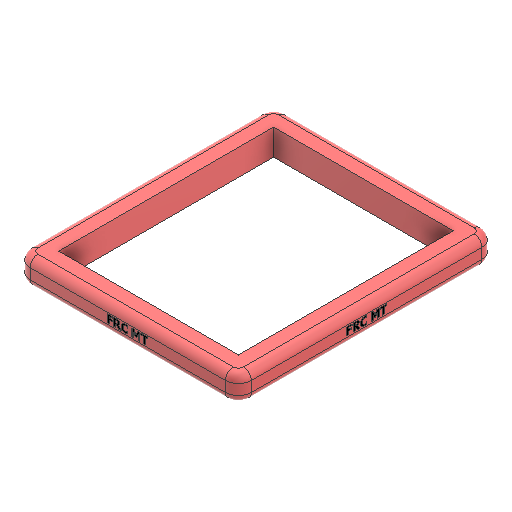
# Autodesk Inventor part: Bumper
Saved by Autodesk Inventor 2027.1 (Build 311270010, 270A)
## iProperties
Created: 2026-08-13
Part Number: Bumper
Material: Genérico
Document SubType Name: Modeling
Designer: djair.oliveira
Density: 1 g/cm^3
Appearance: Padrão
Author: djair.oliveira
Autodesk Inventor part; units mm, degrees
ref_plane "YZ Plane" through (0, 0, 0) normal (1, 0, 0) x (0, 1, 0)
ref_plane "XZ Plane" through (0, 0, 0) normal (0, 1, 0) x (-1, 0, 0)
ref_plane "XY Plane" through (0, 0, 0) normal (0, 0, 1) x (1, 0, 0)
sketch "Esboço1" plane through (0, 0, 0) normal (0, 1, 0) x (-1, 0, 0)
  line L0 (-346.4954, -410.2857) -> (343.3046, -410.2857)
  line L1 (343.3046, -410.2857) -> (343.3046, 414.3883)
  line L2 (343.3046, 414.3883) -> (-346.4954, 414.3883)
  line L3 (-346.4954, 414.3883) -> (-346.4954, -410.2857)
  line L4 (373.3046, -490.2857) -> (-376.4954, -490.2857)
  line L5 (-426.4954, -440.2857) -> (-426.4954, 444.3883)
  line L6 (-376.4954, 494.3883) -> (373.3046, 494.3883)
  line L7 (423.3046, 444.3883) -> (423.3046, -440.2857)
  arc A0 (373.3046, -490.2857) -> (423.3046, -440.2857) centre (373.3046, -440.2857) ccw
  arc A1 (423.3046, 444.3883) -> (373.3046, 494.3883) centre (373.3046, 444.3883) ccw
  arc A2 (-376.4954, 494.3883) -> (-426.4954, 444.3883) centre (-376.4954, 444.3883) ccw
  arc A3 (-426.4954, -440.2857) -> (-376.4954, -490.2857) centre (-376.4954, -440.2857) ccw
  point P0 (0, 0)
  dimension "d4" = 80
  dimension "d5" = 50
  constraints: 16 end point, 8 point on circle, 8 tangent, 4 centre point, 4 parallel, 3 equal radius, 2 perpendicular, 1 horizontal, 3 other
  measures "d4" distance between parallel lines of L0 L4
  measures "d5" radius of A0
extrude "Extrusão1" add sketch "Esboço1" along normal blind 100
fillet "Arredondamento1" radius 30 16 edges at (-408.6599, 100, 479.7436) (1.5954, 100, 494.3883) (411.8508, 100, 479.7436) (426.4954, 100, 2.0513) (411.8508, 100, -475.6411) (1.5954, 100, -490.2857) (-408.6599, 100, -475.6411) (-423.3046, 100, 2.0513) (411.8508, 0, -475.6411) (1.5954, 0, -490.2857) (-408.6599, 0, -475.6411) (-423.3046, 0, 2.0513) (-408.6599, 0, 479.7436) (1.5954, 0, 494.3883) (411.8508, 0, 479.7436) (426.4954, 0, 2.0513)
sketch "Esboço2" plane through (426.4954, 30, -440.2857) normal (1, 0, 0) x (0, 0, -1)
  line L0 (-521.7524, 35.8457) -> (-358.819, 35.8457) construction
  line L1 (-358.819, 35.8457) -> (-358.819, 4.1543) construction
  line L2 (-358.819, 4.1543) -> (-521.7524, 4.1543) construction
  line L3 (-521.7524, 4.1543) -> (-521.7524, 35.8457) construction
  line L4 (-498.5595, 29.5491) -> (-511.1527, 29.5491)
  line L5 (-511.1527, 29.5491) -> (-511.1527, 23.8846)
  line L6 (-511.1527, 23.8846) -> (-499.5563, 23.8846)
  line L7 (-499.5563, 23.8846) -> (-499.5563, 18.1715)
  line L8 (-499.5563, 18.1715) -> (-511.1527, 18.1715)
  line L9 (-511.1527, 18.1715) -> (-511.1527, 5.2623)
  line L10 (-511.1527, 5.2623) -> (-518.6406, 5.2623)
  line L11 (-518.6406, 5.2623) -> (-518.6406, 35.2623)
  line L12 (-518.6406, 35.2623) -> (-498.5595, 35.2623)
  line L13 (-498.5595, 35.2623) -> (-498.5595, 29.5491)
  line L14 (-466.955, 5.2623) -> (-476.1203, 5.2623)
  line L15 (-476.1203, 5.2623) -> (-484.459, 16.2752)
  line L16 (-484.459, 16.2752) -> (-487.1819, 16.2752)
  line L17 (-487.1819, 16.2752) -> (-487.1819, 5.2623)
  line L18 (-487.1819, 5.2623) -> (-494.6697, 5.2623)
  line L19 (-494.6697, 5.2623) -> (-494.6697, 35.2623)
  line L20 (-494.6697, 35.2623) -> (-482.6114, 35.2623)
  spline S0 degree 2 poles (-482.6114, 35.2623) (-480.1073, 35.2623) (-476.412, 34.6302) (-474.8318, 33.6577) knots 0 0 0 1 2 2 2
  spline S1 degree 2 poles (-474.8318, 33.6577) (-473.2273, 32.6367) (-471.331, 29.4519) (-471.331, 27.0208) knots 0 0 0 1 2 2 2
  spline S2 degree 2 poles (-471.331, 27.0208) (-471.331, 23.5929) (-474.4428, 19.2898) (-477.0441, 18.0256) knots 0 0 0 1 2 2 2
  line L21 (-477.0441, 18.0256) -> (-466.955, 5.2623)
  spline S3 degree 2 poles (-479.062, 26.0726) (-479.062, 27.2153) (-479.9372, 28.8441) (-480.9339, 29.2817) knots 0 0 0 1 2 2 2
  spline S4 degree 2 poles (-480.9339, 29.2817) (-481.639, 29.5735) (-483.365, 29.7436) (-484.6535, 29.7436) knots 0 0 0 1 2 2 2
  line L22 (-484.6535, 29.7436) -> (-487.1819, 29.7436)
  line L23 (-487.1819, 29.7436) -> (-487.1819, 21.6723)
  line L24 (-487.1819, 21.6723) -> (-485.0182, 21.6723)
  spline S5 degree 2 poles (-485.0182, 21.6723) (-483.4623, 21.6723) (-481.25, 22.0613) (-480.4963, 22.6691) knots 0 0 0 1 2 2 2
  spline S6 degree 2 poles (-480.4963, 22.6691) (-479.767, 23.2525) (-479.062, 24.8085) (-479.062, 26.0726) knots 0 0 0 1 2 2 2
  spline S7 degree 2 poles (-451.7848, 4.6788) (-458.5433, 4.6788) (-466.4688, 12.8474) (-466.4688, 20.238) knots 0 0 0 1 2 2 2
  spline S8 degree 2 poles (-466.4688, 20.238) (-466.4688, 27.3611) (-458.519, 35.8457) (-451.7605, 35.8457) knots 0 0 0 1 2 2 2
  spline S9 degree 2 poles (-451.7605, 35.8457) (-449.9858, 35.8457) (-447.1171, 35.4324) (-445.8043, 35.0921) knots 0 0 0 1 2 2 2
  spline S10 degree 2 poles (-445.8043, 35.0921) (-444.7832, 34.776) (-442.3764, 33.7307) (-441.6227, 33.3417) knots 0 0 0 1 2 2 2
  line L25 (-441.6227, 33.3417) -> (-441.6227, 26.1942)
  line L26 (-441.6227, 26.1942) -> (-442.3764, 26.1942)
  spline S11 degree 2 poles (-442.3764, 26.1942) (-442.9355, 26.6804) (-444.5887, 28.0418) (-445.6341, 28.6739) knots 0 0 0 1 2 2 2
  spline S12 degree 2 poles (-445.6341, 28.6739) (-446.6795, 29.3303) (-449.1835, 30.2299) (-450.5693, 30.2299) knots 0 0 0 1 2 2 2
  spline S13 degree 2 poles (-450.5693, 30.2299) (-452.1981, 30.2299) (-454.8966, 29.2088) (-456.1365, 27.9203) knots 0 0 0 1 2 2 2
  spline S14 degree 2 poles (-456.1365, 27.9203) (-457.2548, 26.7777) (-458.6892, 22.8636) (-458.6892, 20.2136) knots 0 0 0 1 2 2 2
  spline S15 degree 2 poles (-458.6892, 20.2136) (-458.6892, 17.4179) (-457.2062, 13.601) (-455.9907, 12.4341) knots 0 0 0 1 2 2 2
  spline S16 degree 2 poles (-455.9907, 12.4341) (-454.8237, 11.2914) (-451.955, 10.2947) (-450.5206, 10.2947) knots 0 0 0 1 2 2 2
  spline S17 degree 2 poles (-450.5206, 10.2947) (-449.0377, 10.2947) (-446.3391, 11.2914) (-445.4153, 11.8992) knots 0 0 0 1 2 2 2
  spline S18 degree 2 poles (-445.4153, 11.8992) (-444.3942, 12.507) (-442.8626, 13.7955) (-442.3035, 14.306) knots 0 0 0 1 2 2 2
  line L27 (-442.3035, 14.306) -> (-441.6227, 14.306)
  line L28 (-441.6227, 14.306) -> (-441.6227, 7.2558)
  spline S19 degree 2 poles (-441.6227, 7.2558) (-442.4493, 6.8668) (-444.613, 5.8944) (-445.78, 5.554) knots 0 0 0 1 2 2 2
  spline S20 degree 2 poles (-445.78, 5.554) (-447.19, 5.1164) (-449.6454, 4.6788) (-451.7848, 4.6788) knots 0 0 0 1 2 2 2
  line L29 (-394.459, 5.2623) -> (-401.9469, 5.2623)
  line L30 (-401.9469, 5.2623) -> (-401.9469, 25.1488)
  line L31 (-401.9469, 25.1488) -> (-407.3926, 12.3125)
  line L32 (-407.3926, 12.3125) -> (-412.5466, 12.3125)
  line L33 (-412.5466, 12.3125) -> (-417.9923, 25.1488)
  line L34 (-417.9923, 25.1488) -> (-417.9923, 5.2623)
  line L35 (-417.9923, 5.2623) -> (-425.0911, 5.2623)
  line L36 (-425.0911, 5.2623) -> (-425.0911, 35.2623)
  line L37 (-425.0911, 35.2623) -> (-416.412, 35.2623)
  line L38 (-416.412, 35.2623) -> (-409.7508, 20.4568)
  line L39 (-409.7508, 20.4568) -> (-403.1381, 35.2623)
  line L40 (-403.1381, 35.2623) -> (-394.459, 35.2623)
  line L41 (-394.459, 35.2623) -> (-394.459, 5.2623)
  line L42 (-382.4736, 5.2623) -> (-382.4736, 29.5491)
  line L43 (-382.4736, 29.5491) -> (-391.3472, 29.5491)
  line L44 (-391.3472, 29.5491) -> (-391.3472, 35.2623)
  line L45 (-391.3472, 35.2623) -> (-366.0636, 35.2623)
  line L46 (-366.0636, 35.2623) -> (-366.0636, 29.5491)
  line L47 (-366.0636, 29.5491) -> (-374.9372, 29.5491)
  line L48 (-374.9372, 29.5491) -> (-374.9372, 5.2623)
  line L49 (-374.9372, 5.2623) -> (-382.4736, 5.2623)
  point P0 (-440.2857, -30)
  point P1 (-440.2857, 35.8457)
  point P2 (-358.819, 20)
  dimension "d9" = 0
  dimension "d10" = 50
  constraints: 2 midpoint, 2 other
  measures "d9" horizontal distance of point (-440.286, -30) point (-440.286, 35.846)
  measures "d10" vertical distance of point (-358.819, 20) point (-440.286, -30)
extrude "Extrusão2" cut sketch "Esboço2" against normal blind 0.1
sketch "Esboço3" plane through (376.4954, 30, -490.2857) normal (0, 0, -1) x (-1, 0, 0)
  line L0 (298.952, 35.0044) -> (454.0389, 35.0044) construction
  line L1 (454.0389, 35.0044) -> (454.0389, 4.9956) construction
  line L2 (454.0389, 4.9956) -> (298.952, 4.9956) construction
  line L3 (298.952, 4.9956) -> (298.952, 35.0044) construction
  line L4 (322.1449, 28.7078) -> (309.5517, 28.7078)
  line L5 (309.5517, 28.7078) -> (309.5517, 23.0433)
  line L6 (309.5517, 23.0433) -> (321.1481, 23.0433)
  line L7 (321.1481, 23.0433) -> (321.1481, 17.3301)
  line L8 (321.1481, 17.3301) -> (309.5517, 17.3301)
  line L9 (309.5517, 17.3301) -> (309.5517, 4.4209)
  line L10 (309.5517, 4.4209) -> (302.0638, 4.4209)
  line L11 (302.0638, 4.4209) -> (302.0638, 34.4209)
  line L12 (302.0638, 34.4209) -> (322.1449, 34.4209)
  line L13 (322.1449, 34.4209) -> (322.1449, 28.7078)
  line L14 (353.7494, 4.4209) -> (344.5841, 4.4209)
  line L15 (344.5841, 4.4209) -> (336.2454, 15.4339)
  line L16 (336.2454, 15.4339) -> (333.5225, 15.4339)
  line L17 (333.5225, 15.4339) -> (333.5225, 4.4209)
  line L18 (333.5225, 4.4209) -> (326.0347, 4.4209)
  line L19 (326.0347, 4.4209) -> (326.0347, 34.4209)
  line L20 (326.0347, 34.4209) -> (338.093, 34.4209)
  spline S0 degree 2 poles (338.093, 34.4209) (340.5971, 34.4209) (344.2924, 33.7888) (345.8726, 32.8164) knots 0 0 0 1 2 2 2
  spline S1 degree 2 poles (345.8726, 32.8164) (347.4771, 31.7953) (349.3734, 28.6105) (349.3734, 26.1794) knots 0 0 0 1 2 2 2
  spline S2 degree 2 poles (349.3734, 26.1794) (349.3734, 22.7515) (346.2616, 18.4485) (343.6603, 17.1843) knots 0 0 0 1 2 2 2
  line L21 (343.6603, 17.1843) -> (353.7494, 4.4209)
  spline S3 degree 2 poles (341.6425, 25.2313) (341.6425, 26.3739) (340.7673, 28.0028) (339.7705, 28.4404) knots 0 0 0 1 2 2 2
  spline S4 degree 2 poles (339.7705, 28.4404) (339.0655, 28.7321) (337.3394, 28.9023) (336.0509, 28.9023) knots 0 0 0 1 2 2 2
  line L22 (336.0509, 28.9023) -> (333.5225, 28.9023)
  line L23 (333.5225, 28.9023) -> (333.5225, 20.831)
  line L24 (333.5225, 20.831) -> (335.6862, 20.831)
  spline S5 degree 2 poles (335.6862, 20.831) (337.2421, 20.831) (339.4544, 21.2199) (340.2081, 21.8277) knots 0 0 0 1 2 2 2
  spline S6 degree 2 poles (340.2081, 21.8277) (340.9374, 22.4112) (341.6425, 23.9671) (341.6425, 25.2313) knots 0 0 0 1 2 2 2
  spline S7 degree 2 poles (368.9196, 3.8374) (362.1611, 3.8374) (354.2356, 12.006) (354.2356, 19.3966) knots 0 0 0 1 2 2 2
  spline S8 degree 2 poles (354.2356, 19.3966) (354.2356, 26.5198) (362.1854, 35.0044) (368.9439, 35.0044) knots 0 0 0 1 2 2 2
  spline S9 degree 2 poles (368.9439, 35.0044) (370.7186, 35.0044) (373.5873, 34.5911) (374.9002, 34.2507) knots 0 0 0 1 2 2 2
  spline S10 degree 2 poles (374.9002, 34.2507) (375.9212, 33.9347) (378.328, 32.8893) (379.0817, 32.5003) knots 0 0 0 1 2 2 2
  line L25 (379.0817, 32.5003) -> (379.0817, 25.3528)
  line L26 (379.0817, 25.3528) -> (378.328, 25.3528)
  spline S11 degree 2 poles (378.328, 25.3528) (377.7689, 25.8391) (376.1157, 27.2005) (375.0703, 27.8326) knots 0 0 0 1 2 2 2
  spline S12 degree 2 poles (375.0703, 27.8326) (374.0249, 28.489) (371.5209, 29.3885) (370.1352, 29.3885) knots 0 0 0 1 2 2 2
  spline S13 degree 2 poles (370.1352, 29.3885) (368.5063, 29.3885) (365.8078, 28.3674) (364.5679, 27.0789) knots 0 0 0 1 2 2 2
  spline S14 degree 2 poles (364.5679, 27.0789) (363.4496, 25.9363) (362.0152, 22.0222) (362.0152, 19.3723) knots 0 0 0 1 2 2 2
  spline S15 degree 2 poles (362.0152, 19.3723) (362.0152, 16.5765) (363.4982, 12.7596) (364.7138, 11.5927) knots 0 0 0 1 2 2 2
  spline S16 degree 2 poles (364.7138, 11.5927) (365.8807, 10.4501) (368.7494, 9.4533) (370.1838, 9.4533) knots 0 0 0 1 2 2 2
  spline S17 degree 2 poles (370.1838, 9.4533) (371.6668, 9.4533) (374.3653, 10.4501) (375.2891, 11.0579) knots 0 0 0 1 2 2 2
  spline S18 degree 2 poles (375.2891, 11.0579) (376.3102, 11.6656) (377.8418, 12.9541) (378.401, 13.4647) knots 0 0 0 1 2 2 2
  line L27 (378.401, 13.4647) -> (379.0817, 13.4647)
  line L28 (379.0817, 13.4647) -> (379.0817, 6.4144)
  spline S19 degree 2 poles (379.0817, 6.4144) (378.2551, 6.0254) (376.0914, 5.053) (374.9245, 4.7126) knots 0 0 0 1 2 2 2
  spline S20 degree 2 poles (374.9245, 4.7126) (373.5144, 4.275) (371.059, 3.8374) (368.9196, 3.8374) knots 0 0 0 1 2 2 2
  line L29 (426.2454, 4.4209) -> (418.7575, 4.4209)
  line L30 (418.7575, 4.4209) -> (418.7575, 24.3075)
  line L31 (418.7575, 24.3075) -> (413.3118, 11.4711)
  line L32 (413.3118, 11.4711) -> (408.1579, 11.4711)
  line L33 (408.1579, 11.4711) -> (402.7121, 24.3075)
  line L34 (402.7121, 24.3075) -> (402.7121, 4.4209)
  line L35 (402.7121, 4.4209) -> (395.6133, 4.4209)
  line L36 (395.6133, 4.4209) -> (395.6133, 34.4209)
  line L37 (395.6133, 34.4209) -> (404.2924, 34.4209)
  line L38 (404.2924, 34.4209) -> (410.9536, 19.6154)
  line L39 (410.9536, 19.6154) -> (417.5663, 34.4209)
  line L40 (417.5663, 34.4209) -> (426.2454, 34.4209)
  line L41 (426.2454, 34.4209) -> (426.2454, 4.4209)
  line L42 (438.2308, 4.4209) -> (438.2308, 28.7078)
  line L43 (438.2308, 28.7078) -> (429.3572, 28.7078)
  line L44 (429.3572, 28.7078) -> (429.3572, 34.4209)
  line L45 (429.3572, 34.4209) -> (454.6408, 34.4209)
  line L46 (454.6408, 34.4209) -> (454.6408, 28.7078)
  line L47 (454.6408, 28.7078) -> (445.7673, 28.7078)
  line L48 (445.7673, 28.7078) -> (445.7673, 4.4209)
  line L49 (445.7673, 4.4209) -> (438.2308, 4.4209)
  point P0 (376.4954, -30)
  point P1 (376.4954, 35.0044)
  point P2 (454.0389, 20)
  dimension "d14" = 0
  dimension "d15" = 50
  constraints: 2 midpoint, 2 other
  measures "d14" horizontal distance of point (376.495, 35.004) point (376.495, -30)
  measures "d15" vertical distance of point (454.039, 20) point (376.495, -30)
extrude "Extrusão3" cut sketch "Esboço3" against normal blind 0.1
sketch "Esboço4" plane through (-423.3046, 30, 444.3883) normal (-1, 0, 0) x (0, 0, 1)
  line L0 (-522.2327, 35.6146) -> (-366.5439, 35.6146) construction
  line L1 (-366.5439, 35.6146) -> (-366.5439, 4.3854) construction
  line L2 (-366.5439, 4.3854) -> (-522.2327, 4.3854) construction
  line L3 (-522.2327, 4.3854) -> (-522.2327, 35.6146) construction
  line L4 (-499.0398, 29.318) -> (-511.633, 29.318)
  line L5 (-511.633, 29.318) -> (-511.633, 23.6535)
  line L6 (-511.633, 23.6535) -> (-500.0366, 23.6535)
  line L7 (-500.0366, 23.6535) -> (-500.0366, 17.9404)
  line L8 (-500.0366, 17.9404) -> (-511.633, 17.9404)
  line L9 (-511.633, 17.9404) -> (-511.633, 5.0311)
  line L10 (-511.633, 5.0311) -> (-519.1209, 5.0311)
  line L11 (-519.1209, 5.0311) -> (-519.1209, 35.0311)
  line L12 (-519.1209, 35.0311) -> (-499.0398, 35.0311)
  line L13 (-499.0398, 35.0311) -> (-499.0398, 29.318)
  line L14 (-467.4353, 5.0311) -> (-476.6006, 5.0311)
  line L15 (-476.6006, 5.0311) -> (-484.9393, 16.0441)
  line L16 (-484.9393, 16.0441) -> (-487.6622, 16.0441)
  line L17 (-487.6622, 16.0441) -> (-487.6622, 5.0311)
  line L18 (-487.6622, 5.0311) -> (-495.15, 5.0311)
  line L19 (-495.15, 5.0311) -> (-495.15, 35.0311)
  line L20 (-495.15, 35.0311) -> (-483.0917, 35.0311)
  spline S0 degree 2 poles (-483.0917, 35.0311) (-480.5876, 35.0311) (-476.8923, 34.399) (-475.3121, 33.4266) knots 0 0 0 1 2 2 2
  spline S1 degree 2 poles (-475.3121, 33.4266) (-473.7076, 32.4055) (-471.8113, 29.2208) (-471.8113, 26.7896) knots 0 0 0 1 2 2 2
  spline S2 degree 2 poles (-471.8113, 26.7896) (-471.8113, 23.3618) (-474.9231, 19.0587) (-477.5244, 17.7945) knots 0 0 0 1 2 2 2
  line L21 (-477.5244, 17.7945) -> (-467.4353, 5.0311)
  spline S3 degree 2 poles (-479.5423, 25.8415) (-479.5423, 26.9841) (-480.4175, 28.613) (-481.4142, 29.0506) knots 0 0 0 1 2 2 2
  spline S4 degree 2 poles (-481.4142, 29.0506) (-482.1192, 29.3423) (-483.8453, 29.5125) (-485.1338, 29.5125) knots 0 0 0 1 2 2 2
  line L22 (-485.1338, 29.5125) -> (-487.6622, 29.5125)
  line L23 (-487.6622, 29.5125) -> (-487.6622, 21.4412)
  line L24 (-487.6622, 21.4412) -> (-485.4985, 21.4412)
  spline S5 degree 2 poles (-485.4985, 21.4412) (-483.9426, 21.4412) (-481.7303, 21.8302) (-480.9766, 22.4379) knots 0 0 0 1 2 2 2
  spline S6 degree 2 poles (-480.9766, 22.4379) (-480.2473, 23.0214) (-479.5423, 24.5773) (-479.5423, 25.8415) knots 0 0 0 1 2 2 2
  spline S7 degree 2 poles (-452.2651, 4.4477) (-459.0236, 4.4477) (-466.9491, 12.6162) (-466.9491, 20.0068) knots 0 0 0 1 2 2 2
  spline S8 degree 2 poles (-466.9491, 20.0068) (-466.9491, 27.13) (-458.9993, 35.6146) (-452.2408, 35.6146) knots 0 0 0 1 2 2 2
  spline S9 degree 2 poles (-452.2408, 35.6146) (-450.4661, 35.6146) (-447.5974, 35.2013) (-446.2846, 34.861) knots 0 0 0 1 2 2 2
  spline S10 degree 2 poles (-446.2846, 34.861) (-445.2635, 34.5449) (-442.8567, 33.4995) (-442.103, 33.1105) knots 0 0 0 1 2 2 2
  line L25 (-442.103, 33.1105) -> (-442.103, 25.9631)
  line L26 (-442.103, 25.9631) -> (-442.8567, 25.9631)
  spline S11 degree 2 poles (-442.8567, 25.9631) (-443.4158, 26.4493) (-445.069, 27.8107) (-446.1144, 28.4428) knots 0 0 0 1 2 2 2
  spline S12 degree 2 poles (-446.1144, 28.4428) (-447.1598, 29.0992) (-449.6638, 29.9987) (-451.0495, 29.9987) knots 0 0 0 1 2 2 2
  spline S13 degree 2 poles (-451.0495, 29.9987) (-452.6784, 29.9987) (-455.3769, 28.9776) (-456.6168, 27.6892) knots 0 0 0 1 2 2 2
  spline S14 degree 2 poles (-456.6168, 27.6892) (-457.7351, 26.5465) (-459.1695, 22.6324) (-459.1695, 19.9825) knots 0 0 0 1 2 2 2
  spline S15 degree 2 poles (-459.1695, 19.9825) (-459.1695, 17.1867) (-457.6865, 13.3699) (-456.4709, 12.2029) knots 0 0 0 1 2 2 2
  spline S16 degree 2 poles (-456.4709, 12.2029) (-455.304, 11.0603) (-452.4353, 10.0635) (-451.0009, 10.0635) knots 0 0 0 1 2 2 2
  spline S17 degree 2 poles (-451.0009, 10.0635) (-449.5179, 10.0635) (-446.8194, 11.0603) (-445.8956, 11.6681) knots 0 0 0 1 2 2 2
  spline S18 degree 2 poles (-445.8956, 11.6681) (-444.8745, 12.2759) (-443.3429, 13.5644) (-442.7837, 14.0749) knots 0 0 0 1 2 2 2
  line L27 (-442.7837, 14.0749) -> (-442.103, 14.0749)
  line L28 (-442.103, 14.0749) -> (-442.103, 7.0246)
  spline S19 degree 2 poles (-442.103, 7.0246) (-442.9296, 6.6357) (-445.0933, 5.6632) (-446.2602, 5.3229) knots 0 0 0 1 2 2 2
  spline S20 degree 2 poles (-446.2602, 5.3229) (-447.6703, 4.8853) (-450.1257, 4.4477) (-452.2651, 4.4477) knots 0 0 0 1 2 2 2
  line L29 (-394.9393, 5.0311) -> (-402.4272, 5.0311)
  line L30 (-402.4272, 5.0311) -> (-402.4272, 24.9177)
  line L31 (-402.4272, 24.9177) -> (-407.8729, 12.0814)
  line L32 (-407.8729, 12.0814) -> (-413.0269, 12.0814)
  line L33 (-413.0269, 12.0814) -> (-418.4726, 24.9177)
  line L34 (-418.4726, 24.9177) -> (-418.4726, 5.0311)
  line L35 (-418.4726, 5.0311) -> (-425.5714, 5.0311)
  line L36 (-425.5714, 5.0311) -> (-425.5714, 35.0311)
  line L37 (-425.5714, 35.0311) -> (-416.8923, 35.0311)
  line L38 (-416.8923, 35.0311) -> (-410.2311, 20.2256)
  line L39 (-410.2311, 20.2256) -> (-403.6184, 35.0311)
  line L40 (-403.6184, 35.0311) -> (-394.9393, 35.0311)
  line L41 (-394.9393, 35.0311) -> (-394.9393, 5.0311)
  line L42 (-382.9539, 5.0311) -> (-382.9539, 29.318)
  line L43 (-382.9539, 29.318) -> (-391.8275, 29.318)
  line L44 (-391.8275, 29.318) -> (-391.8275, 35.0311)
  line L45 (-391.8275, 35.0311) -> (-366.5439, 35.0311)
  line L46 (-366.5439, 35.0311) -> (-366.5439, 29.318)
  line L47 (-366.5439, 29.318) -> (-375.4175, 29.318)
  line L48 (-375.4175, 29.318) -> (-375.4175, 5.0311)
  line L49 (-375.4175, 5.0311) -> (-382.9539, 5.0311)
  point P0 (-444.3883, -30)
  point P1 (-444.3883, 35.6146)
  point P2 (-366.5439, 20)
  dimension "d18" = 0
  dimension "d19" = 50
  constraints: 2 midpoint, 2 other
  measures "d18" horizontal distance of point (-444.388, 35.615) point (-444.388, -30)
  measures "d19" vertical distance of point (-366.544, 20) point (-444.388, -30)
extrude "Extrusão4" cut sketch "Esboço4" against normal blind 0.1
sketch "Esboço5" plane through (-373.3046, 30, 494.3883) normal (0, 0, 1) x (1, 0, 0)
  line L0 (294.6469, 35.8182) -> (451.9622, 35.8182) construction
  line L1 (451.9622, 35.8182) -> (451.9622, 4.1818) construction
  line L2 (451.9622, 4.1818) -> (294.6469, 4.1818) construction
  line L3 (294.6469, 4.1818) -> (294.6469, 35.8182) construction
  line L4 (317.8397, 29.5216) -> (305.2465, 29.5216)
  line L5 (305.2465, 29.5216) -> (305.2465, 23.8571)
  line L6 (305.2465, 23.8571) -> (316.843, 23.8571)
  line L7 (316.843, 23.8571) -> (316.843, 18.144)
  line L8 (316.843, 18.144) -> (305.2465, 18.144)
  line L9 (305.2465, 18.144) -> (305.2465, 5.2347)
  line L10 (305.2465, 5.2347) -> (297.7587, 5.2347)
  line L11 (297.7587, 5.2347) -> (297.7587, 35.2347)
  line L12 (297.7587, 35.2347) -> (317.8397, 35.2347)
  line L13 (317.8397, 35.2347) -> (317.8397, 29.5216)
  line L14 (349.4443, 5.2347) -> (340.279, 5.2347)
  line L15 (340.279, 5.2347) -> (331.9402, 16.2477)
  line L16 (331.9402, 16.2477) -> (329.2174, 16.2477)
  line L17 (329.2174, 16.2477) -> (329.2174, 5.2347)
  line L18 (329.2174, 5.2347) -> (321.7295, 5.2347)
  line L19 (321.7295, 5.2347) -> (321.7295, 35.2347)
  line L20 (321.7295, 35.2347) -> (333.7879, 35.2347)
  spline S0 degree 2 poles (333.7879, 35.2347) (336.2919, 35.2347) (339.9872, 34.6027) (341.5675, 33.6302) knots 0 0 0 1 2 2 2
  spline S1 degree 2 poles (341.5675, 33.6302) (343.172, 32.6091) (345.0683, 29.4244) (345.0683, 26.9933) knots 0 0 0 1 2 2 2
  spline S2 degree 2 poles (345.0683, 26.9933) (345.0683, 23.5654) (341.9564, 19.2623) (339.3551, 17.9981) knots 0 0 0 1 2 2 2
  line L21 (339.3551, 17.9981) -> (349.4443, 5.2347)
  spline S3 degree 2 poles (337.3373, 26.0451) (337.3373, 27.1877) (336.4621, 28.8166) (335.4653, 29.2542) knots 0 0 0 1 2 2 2
  spline S4 degree 2 poles (335.4653, 29.2542) (334.7603, 29.5459) (333.0342, 29.7161) (331.7457, 29.7161) knots 0 0 0 1 2 2 2
  line L22 (331.7457, 29.7161) -> (329.2174, 29.7161)
  line L23 (329.2174, 29.7161) -> (329.2174, 21.6448)
  line L24 (329.2174, 21.6448) -> (331.3811, 21.6448)
  spline S5 degree 2 poles (331.3811, 21.6448) (332.937, 21.6448) (335.1493, 22.0338) (335.9029, 22.6416) knots 0 0 0 1 2 2 2
  spline S6 degree 2 poles (335.9029, 22.6416) (336.6323, 23.225) (337.3373, 24.7809) (337.3373, 26.0451) knots 0 0 0 1 2 2 2
  spline S7 degree 2 poles (364.6145, 4.6513) (357.8559, 4.6513) (349.9305, 12.8198) (349.9305, 20.2104) knots 0 0 0 1 2 2 2
  spline S8 degree 2 poles (349.9305, 20.2104) (349.9305, 27.3336) (357.8803, 35.8182) (364.6388, 35.8182) knots 0 0 0 1 2 2 2
  spline S9 degree 2 poles (364.6388, 35.8182) (366.4135, 35.8182) (369.2822, 35.4049) (370.595, 35.0646) knots 0 0 0 1 2 2 2
  spline S10 degree 2 poles (370.595, 35.0646) (371.6161, 34.7485) (374.0229, 33.7031) (374.7765, 33.3142) knots 0 0 0 1 2 2 2
  line L25 (374.7765, 33.3142) -> (374.7765, 26.1667)
  line L26 (374.7765, 26.1667) -> (374.0229, 26.1667)
  spline S11 degree 2 poles (374.0229, 26.1667) (373.4637, 26.6529) (371.8106, 28.0143) (370.7652, 28.6464) knots 0 0 0 1 2 2 2
  spline S12 degree 2 poles (370.7652, 28.6464) (369.7198, 29.3028) (367.2157, 30.2023) (365.83, 30.2023) knots 0 0 0 1 2 2 2
  spline S13 degree 2 poles (365.83, 30.2023) (364.2012, 30.2023) (361.5026, 29.1813) (360.2628, 27.8928) knots 0 0 0 1 2 2 2
  spline S14 degree 2 poles (360.2628, 27.8928) (359.1444, 26.7501) (357.7101, 22.836) (357.7101, 20.1861) knots 0 0 0 1 2 2 2
  spline S15 degree 2 poles (357.7101, 20.1861) (357.7101, 17.3903) (359.1931, 13.5735) (360.4086, 12.4065) knots 0 0 0 1 2 2 2
  spline S16 degree 2 poles (360.4086, 12.4065) (361.5756, 11.2639) (364.4443, 10.2672) (365.8786, 10.2672) knots 0 0 0 1 2 2 2
  spline S17 degree 2 poles (365.8786, 10.2672) (367.3616, 10.2672) (370.0602, 11.2639) (370.984, 11.8717) knots 0 0 0 1 2 2 2
  spline S18 degree 2 poles (370.984, 11.8717) (372.0051, 12.4795) (373.5367, 13.768) (374.0958, 14.2785) knots 0 0 0 1 2 2 2
  line L27 (374.0958, 14.2785) -> (374.7765, 14.2785)
  line L28 (374.7765, 14.2785) -> (374.7765, 7.2283)
  spline S19 degree 2 poles (374.7765, 7.2283) (373.9499, 6.8393) (371.7863, 5.8668) (370.6193, 5.5265) knots 0 0 0 1 2 2 2
  spline S20 degree 2 poles (370.6193, 5.5265) (369.2093, 5.0889) (366.7538, 4.6513) (364.6145, 4.6513) knots 0 0 0 1 2 2 2
  line L29 (421.9402, 5.2347) -> (414.4524, 5.2347)
  line L30 (414.4524, 5.2347) -> (414.4524, 25.1213)
  line L31 (414.4524, 25.1213) -> (409.0067, 12.285)
  line L32 (409.0067, 12.285) -> (403.8527, 12.285)
  line L33 (403.8527, 12.285) -> (398.407, 25.1213)
  line L34 (398.407, 25.1213) -> (398.407, 5.2347)
  line L35 (398.407, 5.2347) -> (391.3081, 5.2347)
  line L36 (391.3081, 5.2347) -> (391.3081, 35.2347)
  line L37 (391.3081, 35.2347) -> (399.9872, 35.2347)
  line L38 (399.9872, 35.2347) -> (406.6485, 20.4292)
  line L39 (406.6485, 20.4292) -> (413.2611, 35.2347)
  line L40 (413.2611, 35.2347) -> (421.9402, 35.2347)
  line L41 (421.9402, 35.2347) -> (421.9402, 5.2347)
  line L42 (433.9256, 5.2347) -> (433.9256, 29.5216)
  line L43 (433.9256, 29.5216) -> (425.0521, 29.5216)
  line L44 (425.0521, 29.5216) -> (425.0521, 35.2347)
  line L45 (425.0521, 35.2347) -> (450.3357, 35.2347)
  line L46 (450.3357, 35.2347) -> (450.3357, 29.5216)
  line L47 (450.3357, 29.5216) -> (441.4621, 29.5216)
  line L48 (441.4621, 29.5216) -> (441.4621, 5.2347)
  line L49 (441.4621, 5.2347) -> (433.9256, 5.2347)
  point P0 (373.3046, -30)
  point P1 (373.3046, 35.8182)
  point P2 (451.9622, 20)
  dimension "d22" = 0
  dimension "d23" = 50
  constraints: 2 midpoint, 2 other
  measures "d22" horizontal distance of point (373.305, 35.818) point (373.305, -30)
  measures "d23" vertical distance of point (451.962, 20) point (373.305, -30)
extrude "Extrusão5" cut sketch "Esboço5" against normal blind 0.1
